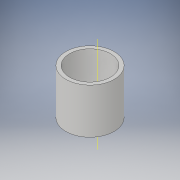
# Autodesk Inventor part: phenolic_liner
Saved by Autodesk Inventor 2017 (Build 210142000, 142)
## iProperties
Created: 2016-10-19
Part Number: phenolic_liner
Material: Generic
Document SubType Name: Modeling
Designer: cflannery
Density: 1 g/cm^3
Appearance: Default
Author: cflannery
Autodesk Inventor part; units mm, degrees
ref_plane "YZ Plane" through (0, 0, 0) normal (1, 0, 0) x (0, 1, 0)
ref_plane "XZ Plane" through (0, 0, 0) normal (0, 1, 0) x (-1, 0, 0)
ref_plane "XY Plane" through (0, 0, 0) normal (0, 0, 1) x (1, 0, 0)
sketch "Sketch1" plane through (0, 0, 0) normal (0, 0, 1) x (1, 0, 0)
  arc A0 (2.8775, -1.3418) -> (0.8218, 3.0668) centre (0, 0) ccw
  line L0 (-17.652, 6.35) -> (-17.652, -31.75)
  line L1 (-17.652, -31.75) -> (-11.302, -31.75)
  line L2 (-11.302, -31.75) -> (2.8775, -1.3418)
  line L3 (-17.652, 6.35) -> (-11.4313, 6.35)
  line L4 (-23.2805, 9.525) -> (0.8218, 3.0668)
  line L5 (-30.352, 9.525) -> (-23.2805, 9.525)
  line L6 (-30.352, 6.35) -> (-30.352, 9.525)
  line L7 (-30.352, 6.35) -> (-20.827, 6.35)
  line L8 (-11.302, -31.75) -> (-24.002, -58.9852)
  line L9 (-17.652, -45.3676) -> (-20.827, -45.3676)
  line L10 (-20.827, 6.35) -> (-20.827, -45.3676)
  line L11 (-30.352, 6.35) -> (-30.352, 3.175)
  line L12 (-30.352, 3.175) -> (-24.002, 3.175)
  line L13 (-24.002, 3.175) -> (-24.002, -52.1764)
  line L14 (-24.002, -52.1764) -> (-20.827, -52.1764)
  line L15 (-28.6587, 3.175) -> (-28.6587, 1.5875)
  line L16 (-28.6587, 1.5875) -> (-30.352, 1.5875)
  line L17 (-30.352, 1.5875) -> (-30.352, -11.1125)
  line L18 (-30.352, -11.1125) -> (-24.002, -11.1125)
  line L19 (-27.177, -39.4764) -> (-27.177, -58.9852)
  line L20 (-27.177, -39.4764) -> (-24.002, -39.4764)
  line L21 (-27.177, -58.9852) -> (-24.002, -58.9852)
  line L22 (-17.652, -6.35) -> (-20.827, -6.35)
  line L23 (0, -72.6873) -> (0, 23.227) projected
  point P0 (6.35, 0)
  dimension "d0" = 6.35
  dimension "d2" = 15
  dimension "d3" = 25
  dimension "d4" = 6.35
  dimension "d5" = 38.1
  dimension "d6" = 6.35
  dimension "d7" = 6.35
  dimension "d15" = 3.175
  dimension "d16" = 3.175
  dimension "d18" = 9.525
  dimension "d20" = 3.175
  dimension "d22" = 3.175
  dimension "d23" = 25
  dimension "d24" = 3.175
  dimension "d25" = 12.7
  dimension "d26" = 1.5875
  dimension "d27" = 1.6933
  dimension "d28" = 3.175
  dimension "d29" = 3.175
  dimension "d30" = 12.7
  dimension "d31" = 3.175
  dimension "d32" = 12.7
  constraints: 46 end point, 9 perpendicular, 7 point on line, 5 horizontal, 5 vertical, 2 coincident, 2 point on circle, 2 tangent, 1 centre point, 1 horizontal alignment, 1 midpoint, 1 parallel, 1 vertical alignment
  measures "d0" diameter of A0
  measures "d2" angle of L3 L4
  measures "d3" angle of L0 L2
  measures "d4" distance of L0.end L1.end
  measures "d5" distance of L0.start L0.end
  measures "d6" distance of point (0, 0) point (6.35, 0)
  measures "d7" vertical distance of point (0, 0) L0.start
  measures "d15" distance of L6.start L5.start
  measures "d16" distance of L0.start L7.end
  measures "d18" distance of L6.start L7.end
  measures "d20" distance between parallel lines of L13 L10
  measures "d22" distance of L9.start L9.end
  measures "d23" angle of L8 L0
  measures "d24" distance of L6.start L11.end
  measures "d25" distance of L16.end L17.end
  measures "d26" distance of L15.start L15.end
  measures "d27" distance of L15.end L16.end
  measures "d28" distance of L13.end L14.end
  measures "d29" distance of L19.start L20.end
  measures "d30" distance of L13.end L20.end
  measures "d31" distance of L19.end L8.end
  measures "d32" distance between parallel lines of L3 L22
revolve "Revolution2" add sketch "Sketch1" angle 360 about axis through (0, -10, 0) along (0, 1, 0) contours L8 L9 L10 L22 L0 L1
body "Solid2"
